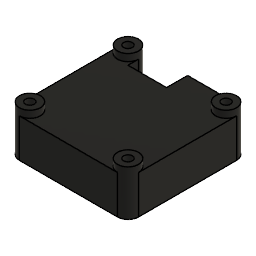
FR Mount (Autodesk Fusion 360 archive; units mm, degrees)
design "Standoff"
part number: 2026-01-23-15-04-41-979
Autodesk Fusion 360 part; units mm, degrees
sketch "Sketch1" plane through (0, 0, 0) normal (0, 0, 1) x (1, 0, 0)
  circle A0 centre (0, 0) radius 1.25
  circle A1 centre (0, 0) radius 3
  circle A2 centre (28, 0) radius 1.25
  circle A3 centre (28, 0) radius 3
  circle A4 centre (0, 28) radius 1.25
  circle A5 centre (0, 28) radius 3
  circle A6 centre (28, 28) radius 1.25
  circle A7 centre (28, 28) radius 3
  dimension "d1" = 2.5
  dimension "d2" = 6
  dimension "d3" = 2.5
  dimension "d4" = 6
  dimension "d5" = 2.5
  dimension "d6" = 6
  dimension "d7" = 28
  dimension "d8" = 28
  dimension "d9" = 2.5
  dimension "d10" = 6
  constraint coincident A0.centre A1.centre
  constraint concentric A0 A1
  constraint concentric A2 A3
  constraint concentric A4 A5
  constraint concentric A6 A7
  measures "d1" diameter of A0
  measures "d2" diameter of A1
  measures "d3" diameter of A2
  measures "d4" diameter of A3
  measures "d5" diameter of A4
  measures "d6" diameter of A5
  measures "d7" distance of A0.centre A4.centre
  measures "d8" distance of A0.centre A2.centre
  measures "d9" diameter of A6
  measures "d10" diameter of A7
sketch "Sketch2" plane through (0, 0, 0) normal (0, 0, -1) x (1, 0, 0)
  circle A0 centre (0, 0) radius 1.25
  circle A1 centre (0, 0) radius 3
  line L0 (0, 3) -> (28, 3)
  line L1 (31, 0) -> (31, -28)
  line L2 (-3, 0) -> (-3, -28)
  line L3 (0, -31) -> (28, -31)
  circle A2 centre (0, -28) radius 3
  circle A3 centre (0, -28) radius 1.25
  circle A4 centre (28, -28) radius 3
  circle A5 centre (28, -28) radius 1.25
  circle A6 centre (28, 0) radius 3
  circle A7 centre (28, 0) radius 1.25
  circle A8 centre (0, 0) radius 3
  line L4 (3, -28) -> (3, -31)
  line L5 (3, -28) -> (3, -25)
  line L6 (3, -25) -> (14, -25)
  line L7 (14, -25) -> (14, -31)
  dimension "d14" = 6
  dimension "d15" = 6
  dimension "d16" = 6
  dimension "d17" = 6
  dimension "d22" = 3
  dimension "d23" = 11
  constraint coincident A1 L0.start
  constraint horizontal L0
  constraint perpendicular L0 L1
  constraint coincident A1 L2.start
  constraint vertical L2
  constraint horizontal L3
  constraint concentric A2 A3
  constraint concentric A4 A5
  constraint concentric A6 A7
  constraint concentric A0 A8
  constraint coincident A2 L4.start
  constraint coincident L3 L4.end
  constraint perpendicular L3 L4
  constraint parallel L4 L5
  constraint perpendicular L4 L6
  constraint midpoint L3 L7.end
  measures "d14" diameter of A2
  measures "d15" diameter of A4
  measures "d16" diameter of A6
  measures "d17" diameter of A8
  measures "d22" distance of L4.start L5.end
  measures "d23" distance of L5.end L6.end
extrude "Extrude3" add sketch "Sketch2" sketch "Sketch1" against normal blind 13 contours A1 A8 | A6 | A4 of sketch 2 contours A5 makes body 1 at (30.9851, 27.7013, 4.3333) makes body 2 at (30.9963, 0.1495, 8.6667) makes body 3 at (2.9963, 0.1495, 8.6667) makes body 4 at (2.9851, 27.7013, 8.6667)
extrude "Extrude4" add sketch "Sketch2" against normal blind 11 contours A1 L0 L1 L2 L3 A2 A4 A6 A8 L5 L6 L7 bodies 1 2 3 4

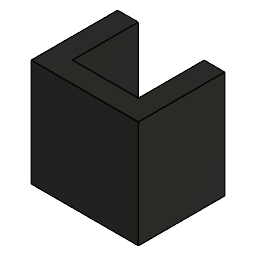
design "Clamp"
part number: 2026-01-01-13-21-08-944
Autodesk Fusion 360 part; units mm, degrees
sketch "Sketch1" plane through (0, 0, 0) normal (0, 0, 1) x (1, 0, 0)
  line L0 (0, 0) -> (0, 25.4)
  line L1 (0, 0) -> (25.4, 0)
  line L2 (25.4, 0) -> (25.4, 25.4)
  line L3 (0, 25.4) -> (-8, 25.4)
  line L4 (-8, -8) -> (33.4, -8)
  line L5 (25.4, 25.4) -> (33.4, 25.4)
  line L6 (-8, 25.4) -> (-8, -8)
  line L7 (33.4, 25.4) -> (33.4, -8)
  dimension "d1" = 25.4
  dimension "d2" = 25.4
  dimension "d3" = 25.4
  dimension "d4" = 8
  dimension "d5" = 8
  dimension "d6" = 8
  constraint coincident L0.start L1.start
  constraint vertical L0
  constraint perpendicular L0 L1
  constraint perpendicular L1 L2
  constraint perpendicular L0 L3
  constraint perpendicular L0 L4
  constraint perpendicular L2 L5
  constraint perpendicular L4 L6
  constraint perpendicular L4 L7
  measures "d1" distance of L0.start L0.end
  measures "d2" distance of L0.start L1.end
  measures "d3" distance of L1.end L2.end
  measures "d4" distance of L0.end L3.end
  measures "d5" distance of L2.end L5.end
  measures "d6" distance of L1 L4
extrude "Extrude3" add sketch "Sketch1" along normal blind 41.4

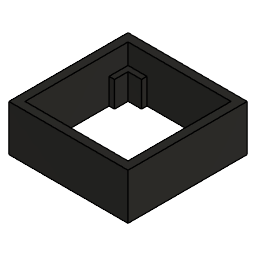
design "Bottom Cover"
part number: 2026-01-23-14-13-38-179
Autodesk Fusion 360 part; units mm, degrees
sketch "Sketch1" plane through (0, 0, 0) normal (0, 0, 1) x (1, 0, 0)
  line L0 (0, 0) -> (44, 0)
  line L1 (44, 0) -> (44, 44)
  line L2 (44, 44) -> (0, 44)
  line L3 (0, 44) -> (0, 0)
  line L4 (3, 3) -> (41, 3)
  line L5 (41, 3) -> (41, 41)
  line L6 (41, 41) -> (3, 41)
  line L7 (3, 41) -> (3, 3)
  dimension "d1" = 44
  dimension "d2" = 44
  dimension "d3" = 3
  dimension "d4" = 3
  dimension "d5" = 3
  dimension "d6" = 3
  constraint horizontal L0
  constraint vertical L1
  constraint horizontal L2
  constraint vertical L3
  constraint coincident L0.start L3.end
  constraint horizontal L4
  constraint vertical L5
  constraint horizontal L6
  constraint vertical L7
  measures "d1" distance of L0.start L0.end
  measures "d2" distance of L0.start L2.end
  measures "d3" distance of L3 L7
  measures "d4" distance of L0 L4
  measures "d5" distance of L1 L5
  measures "d6" distance of L2 L6
sketch "Sketch2" plane through (0, 0, 0) normal (0, 0, -1) x (1, 0, 0)
  line L0 (3, -41) -> (3, -3)
  line L1 (3, -3) -> (41, -3)
  line L2 (41, -3) -> (41, -41)
  line L3 (41, -41) -> (3, -41)
  line L4 (0, 0) -> (0, -44)
  line L5 (0, -44) -> (44, -44)
  line L6 (44, -44) -> (44, 0)
  line L7 (44, 0) -> (0, 0)
  line L8 (3, -10) -> (5, -10)
  line L9 (5, -10) -> (5, -5)
  line L10 (5, -5) -> (10, -5)
  line L11 (10, -5) -> (10, -3)
  line L12 (34, -3) -> (34, -5)
  line L13 (34, -5) -> (39, -5)
  line L14 (39, -5) -> (39, -10)
  line L15 (39, -10) -> (41, -10)
  line L16 (3, -41) -> (3, -34)
  line L17 (3, -34) -> (5, -34)
  line L18 (5, -34) -> (5, -39)
  line L19 (5, -39) -> (10, -39)
  line L20 (10, -39) -> (10, -41)
  line L21 (41, -41) -> (34, -41)
  line L22 (34, -41) -> (34, -39)
  line L23 (34, -39) -> (39, -39)
  line L24 (39, -39) -> (39, -34)
  line L25 (39, -34) -> (41, -34)
  dimension "d9" = 2
  dimension "d10" = 7
  dimension "d11" = 7
  dimension "d12" = 7
  dimension "d13" = 2
  dimension "d14" = 7
  dimension "d15" = 2
  dimension "d16" = 2
  dimension "d17" = 7
  dimension "d18" = 2
  dimension "d19" = 5
  dimension "d20" = 5
  dimension "d21" = 7
  dimension "d22" = 2
  dimension "d23" = 5
  dimension "d24" = 5
  dimension "d25" = 2
  constraint coincident L0 L8.start
  constraint perpendicular L0 L8
  constraint perpendicular L8 L9
  constraint perpendicular L9 L10
  constraint coincident L1 L11.end
  constraint perpendicular L1 L11
  constraint coincident L1 L12.start
  constraint perpendicular L1 L12
  constraint perpendicular L2 L13
  constraint perpendicular L13 L14
  constraint coincident L2 L15.end
  constraint perpendicular L2 L15
  constraint coincident L0.start L3.end
  constraint perpendicular L3 L16
  constraint perpendicular L16 L17
  constraint perpendicular L17 L18
  constraint perpendicular L18 L19
  constraint coincident L3 L20.end
  constraint perpendicular L3 L20
  constraint coincident L2.end L3.start
  constraint perpendicular L2 L21
  constraint perpendicular L21 L22
  constraint perpendicular L2 L23
  constraint perpendicular L21 L24
  constraint perpendicular L24 L25
  measures "d9" distance of L8.start L8.end
  measures "d10" distance of L1 L8
  measures "d11" distance of L0 L11
  measures "d12" distance of L2 L12
  measures "d13" distance of L12.start L12.end
  measures "d14" distance of L1 L15
  measures "d15" distance of L14.end L15.end
  measures "d16" distance of L10.end L11.end
  measures "d17" distance of L0.start L16.end
  measures "d18" distance of L16.end L17.end
  measures "d19" distance of L17.end L18.end
  measures "d20" distance of L18.end L19.end
  measures "d21" distance of L2.end L21.end
  measures "d22" distance of L21.end L22.end
  measures "d23" distance of L22.end L23.end
  measures "d24" distance of L23.end L24.end
  measures "d25" distance of L24.end L25.end
extrude "Extrude3" add sketch "Sketch1" along normal blind 17
extrude "Extrude4" add sketch "Sketch2" against normal blind 9.5 contours L0 L3 L16 L17 L18 L19 L20 | L0 L1 L8 L9 L10 L11 | L2 L3 L21 L22 L23 L24 L25 | L1 L2 L12 L13 L14 L15

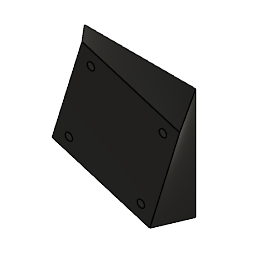
design "FR Bracket"
part number: 2026-01-11-12-51-12-795
Autodesk Fusion 360 part; units mm, degrees
sketch "Sketch1" plane through (0, 0, 0) normal (0, 1, 0) x (1, 0, 0)
  line L0 (0, 0) -> (41.4, 0)
  line L1 (41.4, 0) -> (41.4, -41.4)
  line L2 (41.4, -41.4) -> (0, -41.4)
  line L3 (0, -41.4) -> (0, 0)
  dimension "d1" = 41.4
  dimension "d2" = 41.4
  constraint horizontal L0
  constraint vertical L1
  constraint horizontal L2
  constraint vertical L3
  constraint coincident L0.start L3.end
  measures "d1" distance of L0.start L0.end
  measures "d2" distance of L0.start L2.end
ref_plane "WorkPlane1" through (20.7, -9, 20.7) normal (0, 1, 0) x (1, 0, 0)
sketch "Sketch2" plane through (0, -9, 0) normal (0, 1, 0) x (1, 0, 0)
  line L0 (20.7, -20.7) -> (38.8698, -15.1449)
  line L1 (38.8698, -15.1449) -> (44.4249, -33.3147)
  line L2 (44.4249, -33.3147) -> (8.0853, -44.4249)
  line L3 (8.0853, -44.4249) -> (-3.0249, -8.0853)
  line L4 (-3.0249, -8.0853) -> (33.3147, 3.0249)
  line L5 (33.3147, 3.0249) -> (38.8698, -15.1449)
  point P0 (20.7, -20.7)
  dimension "d41" = 19
  dimension "d42" = 19
  dimension "d43" = 38
  dimension "d44" = 38
  dimension "d45" = 38
  constraint coincident P0 L0.start
  constraint perpendicular L0 L1
  constraint perpendicular L1 L2
  constraint perpendicular L2 L3
  constraint perpendicular L3 L4
  measures "d41" distance of P0 L0.end
  measures "d42" distance of L0.end L1.end
  measures "d43" distance of L1.end L2.end
  measures "d44" distance of L2.end L3.end
  measures "d45" distance of L3.end L4.end
loft "Loft3" add profiles "Sketch2", "Sketch1" section 1 section 2
sketch "Sketch7" plane through (0, -9, 0) normal (0, -1, 0) x (1, 0, 0)
  line L0 (-3.0249, 8.0853) -> (33.3147, -3.0249)
  line L1 (33.3147, -3.0249) -> (44.4249, 33.3147)
  line L2 (44.4249, 33.3147) -> (8.0853, 44.4249)
  line L3 (8.0853, 44.4249) -> (-3.0249, 8.0853)
  line L4 (20.7, 20.7) -> (34.0883, 16.6068)
  circle A0 centre (11.4049, 38.1815) radius 1.35
  circle A1 centre (3.2185, 11.4049) radius 1.35
  circle A2 centre (29.9951, 3.2185) radius 1.35
  circle A3 centre (38.1815, 29.9951) radius 1.35
  dimension "d46" = 14
  dimension "d47" = 14
  dimension "d48" = 28
  dimension "d49" = 28
  dimension "d50" = 28
  dimension "d51" = 2.7
  dimension "d52" = 2.7
  dimension "d53" = 2.7
  dimension "d54" = 2.7
  measures "d46" distance of L4.start L4.end
  measures "d47" distance of L4.end A3.centre
  measures "d48" distance of A0.centre A3.centre
  measures "d49" distance of A0.centre A1.centre
  measures "d50" distance of A1.centre A2.centre
  measures "d51" diameter of A0
  measures "d52" diameter of A1
  measures "d53" diameter of A2
  measures "d54" diameter of A3
extrude "Extrude3" cut sketch "Sketch7" against normal blind 3 contours A0 | A1 | A2 | A3
